gear-encoder-13 v1 (Autodesk Fusion 360 design; units mm, degrees)
description: Spur Gear; Module: 0.3; Num Teeth: 13; Pressure Angle: 20.0; Backlash: 0.00 mm
Autodesk Fusion 360 part; units mm, degrees
sketch "スケッチ1" plane through (0, 0, 0) normal (0, 0, 1) x (1, 0, 0) in component "Spur Gear (13 teeth)"
  circle A0 centre (0, 0) radius 1.5392
  circle A1 centre (0, 0) radius 0.75
extrude "押し出し1" add sketch "スケッチ1" along normal blind 1 in component "Spur Gear (13 teeth)"
sketch "スケッチ2" plane through (0, 0, 0) normal (0, 0, 1) x (1, 0, 0) in component "Spur Gear (13 teeth)"
  spline S0 degree 5 poles (1.8155, -0.248) (1.8168, -0.2481) (1.8192, -0.2484) (1.8228, -0.2487) (1.8276, -0.2489) (1.8337, -0.2489) (1.8398, -0.2487) (1.8458, -0.2484) (1.8519, -0.248) (1.8581, -0.2475) (1.8642, -0.247) (1.8703, -0.2464) (1.8765, -0.2458) (1.8827, -0.245) (1.8888, -0.2441) (1.895, -0.2432) (1.9012, -0.2421) (1.9074, -0.241) (1.9135, -0.2398) (1.9197, -0.2386) (1.9259, -0.2373) (1.9321, -0.2359) (1.9384, -0.2345) (1.9446, -0.233) (1.9508, -0.2314) (1.957, -0.2298) (1.9632, -0.2281) (1.9694, -0.2264) (1.9757, -0.2246) (1.9819, -0.2227) (1.9881, -0.2208) (1.9943, -0.2188) (2.0006, -0.2168) (2.0068, -0.2147) (2.013, -0.2126) (2.0193, -0.2104) (2.0255, -0.2082) (2.0317, -0.2059) (2.038, -0.2035) (2.0442, -0.2011) (2.0504, -0.1987) (2.0566, -0.1962) (2.0629, -0.1936) (2.0691, -0.191) (2.0753, -0.1884) (2.0815, -0.1857) (2.0878, -0.1829) (2.094, -0.1801) (2.1002, -0.1773) (2.1064, -0.1744) (2.1126, -0.1715) (2.1188, -0.1685) (2.125, -0.1654) (2.1312, -0.1624) (2.1374, -0.1592) (2.1436, -0.156) (2.1498, -0.1528) (2.156, -0.1496) (2.1621, -0.1462) (2.1683, -0.1429) (2.1745, -0.1395) (2.1806, -0.136) (2.1868, -0.1325) (2.1929, -0.129) (2.1991, -0.1254) (2.2052, -0.1218) (2.2113, -0.1181) (2.2175, -0.1144) (2.2236, -0.1106) (2.2297, -0.1068) (2.2358, -0.103) (2.2407, -0.0998) (2.2443, -0.0975) (2.2468, -0.0959) (2.248, -0.0951) knots 0 0 0 0 0 0 0.01428571 0.02857143 0.04285714 0.05714286 0.07142857 0.08571429 0.1 0.11428571 0.12857143 0.14285714 0.15714286 0.17142857 0.18571429 0.2 0.21428571 0.22857143 0.24285714 0.25714286 0.27142857 0.28571429 0.3 0.31428571 0.32857143 0.34285714 0.35714286 0.37142857 0.38571429 0.4 0.41428571 0.42857143 0.44285714 0.45714286 0.47142857 0.48571429 0.5 0.51428571 0.52857143 0.54285714 0.55714286 0.57142857 0.58571429 0.6 0.61428571 0.62857143 0.64285714 0.65714286 0.67142857 0.68571429 0.7 0.71428571 0.72857143 0.74285714 0.75714286 0.77142857 0.78571429 0.8 0.81428571 0.82857143 0.84285714 0.85714286 0.87142857 0.88571429 0.9 0.91428571 0.92857143 0.94285714 0.95714286 0.97142857 0.98571429 1 1 1 1 1 1
  spline S1 degree 5 poles (1.8155, 0.248) (1.8168, 0.2481) (1.8192, 0.2484) (1.8228, 0.2487) (1.8276, 0.2489) (1.8337, 0.2489) (1.8398, 0.2487) (1.8458, 0.2484) (1.8519, 0.248) (1.8581, 0.2475) (1.8642, 0.247) (1.8703, 0.2464) (1.8765, 0.2458) (1.8827, 0.245) (1.8888, 0.2441) (1.895, 0.2432) (1.9012, 0.2421) (1.9074, 0.241) (1.9135, 0.2398) (1.9197, 0.2386) (1.9259, 0.2373) (1.9321, 0.2359) (1.9384, 0.2345) (1.9446, 0.233) (1.9508, 0.2314) (1.957, 0.2298) (1.9632, 0.2281) (1.9694, 0.2264) (1.9757, 0.2246) (1.9819, 0.2227) (1.9881, 0.2208) (1.9943, 0.2188) (2.0006, 0.2168) (2.0068, 0.2147) (2.013, 0.2126) (2.0193, 0.2104) (2.0255, 0.2082) (2.0317, 0.2059) (2.038, 0.2035) (2.0442, 0.2011) (2.0504, 0.1987) (2.0566, 0.1962) (2.0629, 0.1936) (2.0691, 0.191) (2.0753, 0.1884) (2.0815, 0.1857) (2.0878, 0.1829) (2.094, 0.1801) (2.1002, 0.1773) (2.1064, 0.1744) (2.1126, 0.1715) (2.1188, 0.1685) (2.125, 0.1654) (2.1312, 0.1624) (2.1374, 0.1592) (2.1436, 0.156) (2.1498, 0.1528) (2.156, 0.1496) (2.1621, 0.1462) (2.1683, 0.1429) (2.1745, 0.1395) (2.1806, 0.136) (2.1868, 0.1325) (2.1929, 0.129) (2.1991, 0.1254) (2.2052, 0.1218) (2.2113, 0.1181) (2.2175, 0.1144) (2.2236, 0.1106) (2.2297, 0.1068) (2.2358, 0.103) (2.2407, 0.0998) (2.2443, 0.0975) (2.2468, 0.0959) (2.248, 0.0951) knots 0 0 0 0 0 0 0.01428571 0.02857143 0.04285714 0.05714286 0.07142857 0.08571429 0.1 0.11428571 0.12857143 0.14285714 0.15714286 0.17142857 0.18571429 0.2 0.21428571 0.22857143 0.24285714 0.25714286 0.27142857 0.28571429 0.3 0.31428571 0.32857143 0.34285714 0.35714286 0.37142857 0.38571429 0.4 0.41428571 0.42857143 0.44285714 0.45714286 0.47142857 0.48571429 0.5 0.51428571 0.52857143 0.54285714 0.55714286 0.57142857 0.58571429 0.6 0.61428571 0.62857143 0.64285714 0.65714286 0.67142857 0.68571429 0.7 0.71428571 0.72857143 0.74285714 0.75714286 0.77142857 0.78571429 0.8 0.81428571 0.82857143 0.84285714 0.85714286 0.87142857 0.88571429 0.9 0.91428571 0.92857143 0.94285714 0.95714286 0.97142857 0.98571429 1 1 1 1 1 1
  arc A0 (2.248, -0.0951) -> (2.248, 0.0951) centre (0, 0) ccw
  line L0 (1.5151, -0.2083) -> (1.8155, -0.248)
  line L1 (1.5151, 0.2083) -> (1.8155, 0.248)
  line L2 (1.5151, -0.2083) -> (1.5151, 0.2083)
  point P0 (1.8456, -0.2484)
  point P1 (1.876, -0.2458)
  point P2 (1.9067, -0.2411)
  point P3 (1.9376, -0.2346)
  point P4 (1.9685, -0.2266)
  point P5 (1.9996, -0.2171)
  point P6 (2.0308, -0.2062)
  point P7 (2.0619, -0.194)
  point P8 (2.0931, -0.1805)
  point P9 (2.1242, -0.1658)
  point P10 (2.1553, -0.1499)
  point P11 (2.1863, -0.1328)
  point P12 (2.2172, -0.1145)
  point P13 (1.8456, 0.2484)
  point P14 (1.876, 0.2458)
  point P15 (1.9067, 0.2411)
  point P16 (1.9376, 0.2346)
  point P17 (1.9685, 0.2266)
  point P18 (1.9996, 0.2171)
  point P19 (2.0308, 0.2062)
  point P20 (2.0619, 0.194)
  point P21 (2.0931, 0.1805)
  point P22 (2.1242, 0.1658)
  point P23 (2.1553, 0.1499)
  point P24 (2.1863, 0.1328)
  point P25 (2.2172, 0.1145)
extrude "押し出し2" add sketch "スケッチ2" along normal blind 1 in component "Spur Gear (13 teeth)"
pattern_circular "C パターン1" count 13 over 360 about axis through (0, 0, 0) along (0, 0, 1) of "押し出し2" in component "Spur Gear (13 teeth)"
sketch "スケッチ3" plane through (0, 0, 0) normal (0, 0, 1) x (1, 0, 0) in component "Spur Gear (13 teeth)"
  circle A0 centre (0, 0) radius 1.95 construction
component "Spur Gear (13 teeth)" placed x (1, 0, 0) y (0, 1, 0) z (0, 0, 1) at (0, 0, 0)
